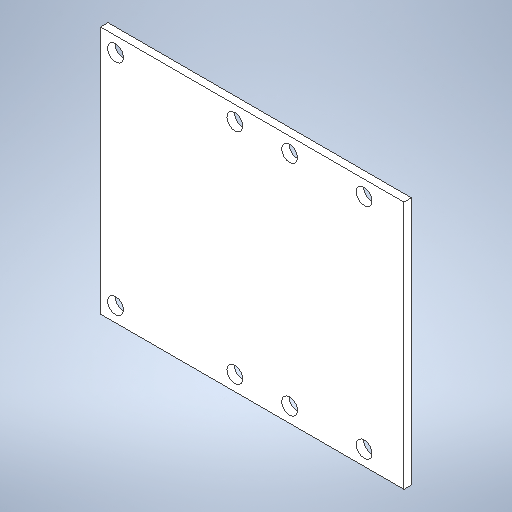
# Autodesk Inventor part: 回収機構天井
Saved by Autodesk Inventor 2026.2 (Build 302298010, 298A)
## iProperties
Created: 2026-05-07
Part Number: 回収機構天井
Material: 一般
Document SubType Name: Modeling
Designer: Yagis
Density: 1 g/cm^3
Appearance: 既定
Author: Yagis
Autodesk Inventor part; units mm, degrees
ref_plane "YZ Plane" through (0, 0, 0) normal (1, 0, 0) x (0, 1, 0)
ref_plane "XZ Plane" through (0, 0, 0) normal (0, 1, 0) x (-1, 0, 0)
ref_plane "XY Plane" through (0, 0, 0) normal (0, 0, 1) x (1, 0, 0)
sketch "スケッチ1" plane through (0, 0, 0) normal (0, 0, 1) x (1, 0, 0)
  line L0 (-30.5, 25) -> (30.5, 25)
  line L1 (30.5, 25) -> (30.5, -25)
  line L2 (30.5, -25) -> (-30.5, -25)
  line L3 (-30.5, -25) -> (-30.5, 25)
  point P0 (0, 0)
  point P1 (-30.5, 0)
  point P2 (0, 25)
  point P3 (-27.5, 22)
  point P4 (7.5, 22)
  point P5 (7.5, -22)
  point P6 (-27.5, -22)
  point P7 (-3.5, -22)
  point P8 (-3.5, 22)
  point P9 (22.5, 22)
  point P10 (22.5, -22)
  dimension "d0" = 50
  dimension "d1" = 61
  dimension "d2" = 35
  dimension "d3" = 44
  dimension "d4" = 3
  dimension "d5" = 3
  dimension "d18" = 44
  dimension "d20" = 22
  dimension "d23" = 26
  dimension "d26" = 11
  constraints: 8 end point, 5 horizontal alignment, 5 vertical alignment, 2 midpoint, 2 parallel, 1 horizontal, 1 perpendicular
  measures "d0" distance of L0.end L1.end
  measures "d1" distance of L0.start L0.end
  measures "d2" distance of point (7.5, 22) point (-27.5, 22)
  measures "d3" distance of point (-27.5, -22) point (-27.5, 22)
  measures "d4" distance from line of L3 point (-27.5, 22)
  measures "d5" distance from line of L0 point (-27.5, 22)
  measures "d18" distance of point (-3.5, -22) point (-3.5, 22)
  measures "d20" vertical distance of point (-3.5, 22) point (0, 0)
  measures "d23" distance of point (-3.5, 22) point (22.5, 22)
  measures "d26" distance of point (-3.5, 22) point (7.5, 22)
extrude "押し出し1" add sketch "スケッチ1" along normal blind 1.5
hole "穴1" at (-27.5, 22, 0) at (7.5, 22, 0) at (7.5, -22, 0) at (-27.5, -22, 0) at (-3.5, -22, 0) at (-3.5, 22, 0) at (22.5, 22, 0) at (22.5, -22, 0) direction (0, 0, 1) diameter 3.2 depth 8.8 tip angle 118
equation "\"d20\" = 0.5 * d18"
